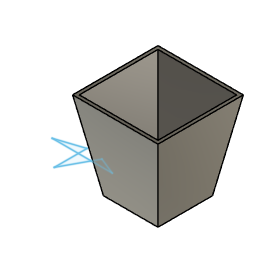
10409김태균_사각통 (Autodesk Fusion 360 design; units mm, degrees)
Autodesk Fusion 360 part; units mm, degrees
sketch "스케치1" plane through (0, 0, 0) normal (0, 0, 1) x (1, 0, 0)
  line L0 (-25, 25) -> (25, 25)
  line L1 (25, 25) -> (25, -25)
  line L2 (25, -25) -> (-25, -25)
  line L3 (-25, -25) -> (-25, 25)
  constraint horizontal L0
  constraint vertical L1
  constraint horizontal L2
  constraint vertical L3
sketch "스케치2" plane through (0, 0, 0) normal (0, 0, 1) x (1, 0, 0)
  line L0 (-54.7462, 3.4053) -> (-38.8986, -3.0124)
  line L1 (-38.8986, -3.0124) -> (-94.0377, -2.8814)
  line L2 (-94.0377, -2.8814) -> (-70, 5)
  line L3 (-70, 5) -> (-70, -25)
  line L4 (-70, -25) -> (-54.7462, 3.4053)
extrude "돌출1" add sketch "스케치1" along normal blind 30 draft 10
extrude "돌출2" add 1 faces at (-10.0966, 10.0966, 30) along direction (0, 0, 1) blind 50 draft 10
shell "쉘1" thickness 3 removed faces 1 at (-13.0354, 13.0354, 80)
